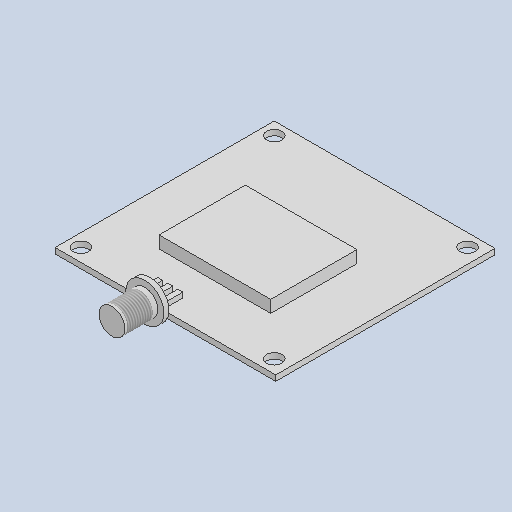
# Autodesk Inventor part: ZED-F9P-02B
Saved by Autodesk Inventor 2025.2 (Build 292293000, 293)
## iProperties
Created: 2025-05-12
Part Number: ZED-F9P-02B
Material: 일반
Document SubType Name: Modeling
Designer: jbhma
Density: 1 g/cm^3
Appearance: 기본값
Author: jbhma
Autodesk Inventor part; units mm, degrees
ref_plane "YZ Plane" through (0, 0, 0) normal (1, 0, 0) x (0, 1, 0)
ref_plane "XZ Plane" through (0, 0, 0) normal (0, 1, 0) x (-1, 0, 0)
ref_plane "XY Plane" through (0, 0, 0) normal (0, 0, 1) x (1, 0, 0)
sketch "스케치1" plane through (0, 0, 0) normal (0, 1, 0) x (-1, 0, 0)
  line L0 (-21.75, -43.2) -> (21.75, -43.2)
  line L1 (21.75, -43.2) -> (21.75, 0)
  line L2 (21.75, 0) -> (-21.75, 0)
  line L3 (-21.75, 0) -> (-21.75, -43.2)
  point P0 (0, 0)
  point P1 (0, 0)
  dimension "d0" = 43.5
  dimension "d1" = 43.2
  constraints: 8 end point, 2 parallel, 1 coincident, 1 horizontal, 1 midpoint, 1 perpendicular
  measures "d0" distance of L2.end L1.end
  measures "d1" distance of L1.end L0.end
extrude "돌출1" add sketch "스케치1" along normal blind 1.1
sketch "스케치2" plane through (0, 1.1, 0) normal (0, 1, 0) x (1, 0, 0)
  line L0 (-21.75, 43.2) -> (-21.75, 0) projected
  line L1 (-21.75, 0) -> (21.75, 0) projected
  line L2 (21.75, 0) -> (21.75, 43.2) projected
  line L3 (21.75, 43.2) -> (-21.75, 43.2) projected
  line L4 (-5.55, 0) -> (-4.55, 0)
  line L5 (-4.55, 0) -> (-4.55, 4)
  line L6 (-4.55, 4) -> (-5.55, 4)
  line L7 (-5.55, 4) -> (-5.55, 0)
  line L8 (-3.55, 0) -> (-2.55, 0)
  line L9 (-2.55, 0) -> (-2.55, 4)
  line L10 (-2.55, 4) -> (-3.55, 4)
  line L11 (-3.55, 4) -> (-3.55, 0)
  line L12 (-1.55, 0) -> (-0.55, 0)
  line L13 (-0.55, 0) -> (-0.55, 4)
  line L14 (-0.55, 4) -> (-1.55, 4)
  line L15 (-1.55, 4) -> (-1.55, 0)
  point P0 (0, 0)
  point P1 (-0.55, 0)
  point P2 (-2.55, 0)
  point P3 (-4.55, 0)
  dimension "d5" = 1
  dimension "d6" = 4
  dimension "d7" = 1
  dimension "d8" = 1
  dimension "d9" = 4
  dimension "d10" = 1
  dimension "d11" = 1
  dimension "d12" = 4
  dimension "d13" = 22.3
  constraints: 24 end point, 6 parallel, 3 horizontal, 3 perpendicular, 3 point on line
  measures "d5" distance of L6.end L5.end
  measures "d6" distance of L5.end L4.end
  measures "d7" distance of L4.end L8.start
  measures "d8" distance of L10.end L9.end
  measures "d9" distance of L9.end L8.end
  measures "d10" distance of L8.end L12.start
  measures "d11" distance of L14.end L13.end
  measures "d12" distance of L13.end L12.end
  measures "d13" distance between parallel lines of L2 L13
extrude "돌출2" add sketch "스케치2" along normal blind 1 contours L7 L6 L5 L1 | L1 L15 L14 L13 | L11 L10 L9 L1
sketch "스케치7" plane through (-21.75, 0, 0) normal (0, 0, 1) x (1, 0, 0)
  line L0 (0, 0) -> (43.5, 0) projected
  line L1 (43.5, 0) -> (43.5, 1.1) projected
  line L2 (21.2, 1.1) -> (43.5, 1.1) projected
  line L3 (21.2, 1.1) -> (21.2, 2.1) projected
  line L4 (20.2, 2.1) -> (21.2, 2.1) projected
  line L5 (20.2, 1.1) -> (20.2, 2.1) projected
  line L6 (19.2, 1.1) -> (20.2, 1.1) projected
  line L7 (19.2, 1.1) -> (19.2, 2.1) projected
  line L8 (18.2, 2.1) -> (19.2, 2.1) projected
  line L9 (18.2, 1.1) -> (18.2, 2.1) projected
  line L10 (17.2, 1.1) -> (18.2, 1.1) projected
  line L11 (17.2, 1.1) -> (17.2, 2.1) projected
  line L12 (16.2, 2.1) -> (17.2, 2.1) projected
  line L13 (16.2, 1.1) -> (16.2, 2.1) projected
  line L14 (0, 1.1) -> (16.2, 1.1) projected
  line L15 (0, 0) -> (0, 1.1) projected
  circle A0 centre (18.7, 1.6) radius 3.75
  point P0 (21.75, 0)
  dimension "d43" = 7.5
  constraints: 1 centre point
  measures "d43" diameter of A0
extrude "돌출7" add sketch "스케치7" along normal blind 1 contours A0 L14 L13 L12 L11 L10 L9 L8 L7 L6 L5 L4 L3 L2 L0 | L0 A0 | A0 L2 L3 L4 L5 L6 L7 L8 L9 L10 L11 L12 L13 L14
sketch "스케치8" plane through (-3.05, 1.6, 1) normal (0, 0, 1) x (1, 0, 0)
  circle A0 centre (0, 0) radius 3.75 projected
  circle A1 centre (0, 0) radius 2.55
  point P0 (3.05, -1.6)
  dimension "d46" = 5.1
  constraints: 1 centre point, 1 coincident
  measures "d46" diameter of A1
extrude "돌출8" add sketch "스케치8" along normal blind 6.5 contours A1
thread "스레드2" size "M5.5x0.5" class "6g" standard "ISO Metric profile" length 5 offset 1
sketch "스케치9" plane through (0, 1.1, 0) normal (0, 1, 0) x (1, 0, 0)
  line L0 (-0.55, 4) -> (-0.55, 0) projected
  line L1 (-0.55, 0) -> (0.6665, 0) projected
  line L2 (0.6665, 0) -> (21.75, 0) projected
  line L3 (21.75, 0) -> (21.75, 43.2) projected
  line L4 (21.75, 43.2) -> (-21.75, 43.2) projected
  line L5 (-21.75, 43.2) -> (-21.75, 0) projected
  line L6 (-21.75, 0) -> (-6.7665, 0) projected
  line L7 (-6.7665, 0) -> (-5.55, 0) projected
  line L8 (-5.55, 0) -> (-5.55, 4) projected
  line L9 (-5.55, 4) -> (-4.55, 4) projected
  line L10 (-4.55, 4) -> (-4.55, 0) projected
  line L11 (-4.55, 0) -> (-3.55, 0) projected
  line L12 (-3.55, 0) -> (-3.55, 4) projected
  line L13 (-3.55, 4) -> (-2.55, 4) projected
  line L14 (-2.55, 4) -> (-2.55, 0) projected
  line L15 (-2.55, 0) -> (-1.55, 0) projected
  line L16 (-1.55, 0) -> (-1.55, 4) projected
  line L17 (-1.55, 4) -> (-0.55, 4) projected
  line L18 (-11.25, 27) -> (10.75, 27)
  line L19 (10.75, 27) -> (10.75, 10)
  line L20 (10.75, 10) -> (-11.25, 10)
  line L21 (-11.25, 10) -> (-11.25, 27)
  point P0 (0, 0)
  dimension "d51" = 22
  dimension "d52" = 17
  dimension "d53" = 10.5
  dimension "d54" = 10
  constraints: 8 end point, 2 parallel, 1 horizontal, 1 perpendicular
  measures "d51" distance of L19.end L20.end
  measures "d52" distance of L18.end L19.end
  measures "d53" distance between parallel lines of L5 L21
  measures "d54" distance between parallel lines of L2 L20
extrude "돌출9" add sketch "스케치9" along normal blind 2.4 contours L18 L19 L20 L21
sketch "스케치11" plane through (0, 1.1, 0) normal (0, 1, 0) x (1, 0, 0)
  circle A0 centre (-19.25, 40.7) radius 1.5
  circle A1 centre (-19.25, 2.6) radius 1.5
  circle A2 centre (18.85, 2.6) radius 1.5
  circle A3 centre (18.85, 40.7) radius 1.5
  line L0 (21.75, 43.2) -> (-21.75, 43.2) projected
  line L1 (-21.75, 43.2) -> (-21.75, 0) projected
  point P0 (0, 0)
  dimension "d71" = 3
  dimension "d72" = 3
  dimension "d73" = 3
  dimension "d74" = 3
  dimension "d75" = 2.5
  dimension "d76" = 2.5
  dimension "d77" = 38.1
  dimension "d78" = 2.5
  dimension "d79" = 38.1
  dimension "d80" = 38.1
  dimension "d81" = 38.1
  dimension "d82" = 2.5
  constraints: 4 centre point
  measures "d71" diameter of A0
  measures "d72" diameter of A1
  measures "d73" diameter of A2
  measures "d74" diameter of A3
  measures "d75" distance from line of L0 A0.centre
  measures "d76" distance from line of L1 A0.centre
  measures "d77" distance of A3.centre A0.centre
  measures "d78" distance from line of L0 A3.centre
  measures "d79" distance of A2.centre A3.centre
  measures "d80" distance of A1.centre A0.centre
  measures "d81" distance of A2.centre A1.centre
  measures "d82" distance from line of L1 A1.centre
extrude "돌출11" cut sketch "스케치11" against normal blind 1.1
